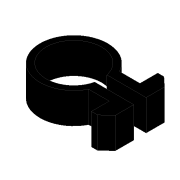
# Autodesk Inventor part: V Slot Clip Wire Holder
Saved by Autodesk Inventor 2020 (Build 240168000, 168)
## iProperties
Created: 2021-09-05
Part Number: V Slot Clip Wire Holder
Material: Generic
Document SubType Name: Modeling
Designer: Coy
Density: 1 g/cm^3
Appearance: Anodized - Black
Author: Coy
Autodesk Inventor part; units mm, degrees
ref_plane "YZ Plane" through (0, 0, 0) normal (1, 0, 0) x (0, 1, 0)
ref_plane "XZ Plane" through (0, 0, 0) normal (0, 1, 0) x (-1, 0, 0)
ref_plane "XY Plane" through (0, 0, 0) normal (0, 0, 1) x (1, 0, 0)
sketch "Sketch1" plane through (0, 0, 0) normal (0, 1, 0) x (-1, 0, 0)
  arc A0 (-4.3875, -1) -> (-4.3875, 1) centre (0, 0) ccw
  line L0 (-10.75, -1) -> (-4.3875, -1)
  line L1 (-8.25, -2.5) -> (-4.899, -2.5)
  line L2 (0, 0) -> (18.2262, 0) construction
  line L3 (-8.25, -2.5) -> (-8.25, -5.4)
  line L4 (-10.75, -1) -> (-10.75, -4)
  line L5 (-8.25, -5.4) -> (-9.25, -5.4)
  line L6 (-9.25, -5.4) -> (-10.75, -4)
  line L7 (-10.75, 1) -> (-4.3875, 1)
  line L8 (-8.25, 2.5) -> (-4.899, 2.5)
  line L9 (-8.25, 2.5) -> (-8.25, 5.4)
  line L10 (-10.75, 1) -> (-10.75, 4)
  line L11 (-8.25, 5.4) -> (-9.25, 5.4)
  line L12 (-9.25, 5.4) -> (-10.75, 4)
  arc A1 (-4.899, -2.5) -> (-4.899, 2.5) centre (0, 0) ccw
  point P0 (-5.692, 1)
  dimension "d0" = 9
  dimension "d3" = 1.5
  dimension "d4" = 1
  dimension "d7" = 3
  dimension "d10" = 4.4
  dimension "d16" = 1
  dimension "d17" = 3.351
  dimension "d18" = 5.5
  dimension "d20" = 2.5
  constraints: 26 end point, 6 symmetric about line, 4 point on circle, 2 centre point, 2 coincident, 1 horizontal, 1 parallel, 1 perpendicular, 1 point on line
  measures "d0" diameter of A0
  measures "d3" distance between parallel lines of L0 L1
  measures "d4" distance from line of point (0, 0) L0
  measures "d7" distance of L0.start L4.end
  measures "d10" distance from line of L0 L3.end
  measures "d16" distance of L3.end L5.end
  measures "d17" distance of L1.start L1.end
  measures "d18" radius of A1
  measures "d20" distance between parallel lines of L3 L4
extrude "Extrusion1" add sketch "Sketch1" along normal blind 5
body "Solid1"
